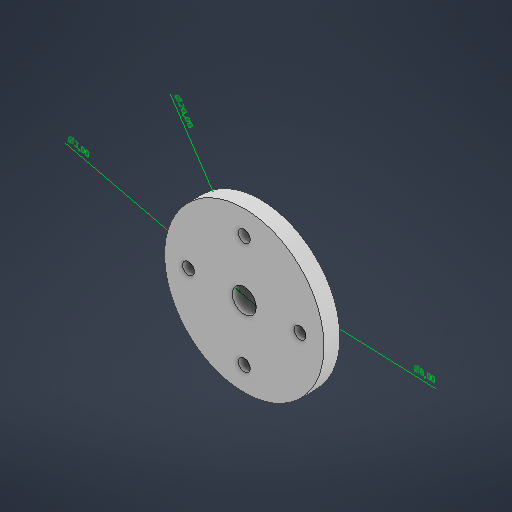
# Autodesk Inventor part: Brida de servo
Saved by Autodesk Inventor 2026 (Build 300175000, 175)
## iProperties
Created: 2025-08-24
Part Number: Brida de servo
Material: Genérico
Document SubType Name: Modeling
Designer: Thomas
Density: 1 g/cm^3
Appearance: Valor por defecto
Author: Thomas
Autodesk Inventor part; units mm, degrees
ref_plane "YZ Plane" through (0, 0, 0) normal (1, 0, 0) x (0, 1, 0)
ref_plane "XZ Plane" through (0, 0, 0) normal (0, 1, 0) x (-1, 0, 0)
ref_plane "XY Plane" through (0, 0, 0) normal (0, 0, 1) x (1, 0, 0)
sketch "Boceto1" plane through (0, 0, 0) normal (1, 0, 0) x (0, 1, 0)
  line L0 (1.5, 0) -> (1.5, -5)
  line L1 (1.5, -5) -> (4, -5)
  line L2 (4, -5) -> (4, -2)
  line L3 (4, -2) -> (10, -2)
  line L4 (10, -2) -> (10, 0)
  line L5 (10, 0) -> (1.5, 0)
  line L6 (0, 0) -> (0, -11.2963)
  line L7 (0, -13.5555) -> (0, 2.2593) projected
  dimension "d0" = 10
  dimension "d1" = 1.5
  dimension "d4" = 4
  dimension "d6" = 2
  dimension "d7" = 5
  constraints: 14 end point, 5 perpendicular, 2 vertical, 1 horizontal alignment
  measures "d0" distance from line of L6.start L4
  measures "d1" distance from line of L0 L6.start
  measures "d4" distance from line of L6.start L2
  measures "d6" distance of L3.end L4.end
  measures "d7" distance of L0.start L0.end
revolve "Revolución1" add sketch "Boceto1" angle 360 about axis through (0, 0, -10) along (0, 0, 1)
sketch "Boceto2" plane through (0, 0, -2) normal (0, 0, -1) x (-1, 0, 0)
  circle A0 centre (0, 7) radius 0.75
  circle A1 centre (-7, 0) radius 0.75
  circle A2 centre (0, -7) radius 0.75
  circle A3 centre (7, 0) radius 0.75
  circle A4 centre (0, 0) radius 7
  dimension "d25" = 14
  dimension "d20" = 1.5
  dimension "d23" = 360
  constraints: 4 centre point, 2 vertical alignment, 1 coincident, 11 other
  measures "d20" diameter of A0
extrude "Extrusión1" cut sketch "Boceto2" against normal through all contours A0 A4 | A4 A0 | A4 A1 | A1 A4 | A4 A3 | A3 A4 | A4 A2 | A2 A4
